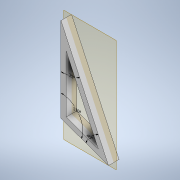
# Autodesk Inventor part: stopForSaltChute
Saved by Autodesk Inventor 2021.1 (Build 251245000, 245)
## iProperties
Created: 2020-09-07
Part Number: stopForSaltChute
Material: Generic
Document SubType Name: Modeling
Designer: robst
Density: 1 g/cm^3
Appearance: Default
Author: robst
Autodesk Inventor part; units mm, degrees
ref_plane "YZ Plane" through (0, 0, 0) normal (1, 0, 0) x (0, 1, 0)
ref_plane "XZ Plane" through (0, 0, 0) normal (0, 1, 0) x (-1, 0, 0)
sketch "Sketch1" plane through (0, 0, 0) normal (0, 0, 1) x (1, 0, 0)
  line L0 (0, 0) -> (0, 152.9054)
  line L1 (0, 152.9054) -> (85.876, -31.2563)
  line L2 (85.876, -31.2563) -> (0, 0)
  dimension "d22" = 45
  dimension "d23" = 110
  dimension "d24" = 203.2
  constraints: 6 end point
  measures "d22" angle of L1 L2
  measures "d23" angle of L2 L0
  measures "d24" distance of L0.end L1.end
extrude "Extrusion1" add sketch "Sketch1" along normal mid plane 19.05
sketch "Sketch2" plane through (0, 0, 0) normal (0, 0, 1) x (1, 0, 0)
  line L0 (9.525, 6.6695) -> (9.525, 109.9409)
  line L1 (9.525, 109.9409) -> (67.5252, -14.4409)
  line L2 (67.5252, -14.4409) -> (9.525, 6.6695)
  line L3 (0, 0) -> (0, 152.9054) projected
  line L4 (0, 152.9054) -> (85.876, -31.2563) projected
  line L5 (85.876, -31.2563) -> (0, 0) projected
  dimension "d4" = 9.525
  dimension "d5" = 9.525
  dimension "d6" = 9.525
  constraints: 6 end point, 3 parallel, 1 vertical, 1 other
  measures "d4" distance between parallel lines of L0 L3
  measures "d5" distance between parallel lines of L1 L4
  measures "d6" distance between parallel lines of L2 L5
extrude "Extrusion2" cut sketch "Sketch2" against normal through all both and the other way through all contours L0 L1 L2
equation "\"d22\" = basicAngle"
equation "\"d23\" = longAngle"
equation "\"d24\" = maxLength"
equation "\"d2\" = width"
equation "\"d4\" = wallThickness"
equation "\"d5\" = wallThickness"
equation "\"d6\" = wallThickness"
equation "\"basicAngle\" = 45deg"
equation "\"maxLength\" = 203.2"
equation "\"wallThickness\" = 9.525"
equation "\"longAngle\" = 110deg"
equation "\"width\" = 19.05"
body "Solid1"
